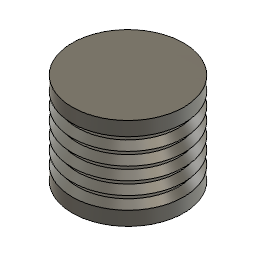
capstan_motor_ed (Autodesk Fusion 360 design; units mm, degrees)
Autodesk Fusion 360 part; units mm, degrees
sketch "Sketch1" plane through (0, 0, 0) normal (0, 1, 0) x (1, 0, 0)
  circle A0 centre (0, 0) radius 10.936
  dimension "d2" = 21.872
  constraint coincident A0.centre origin
  measures "d2" diameter of A0
extrude "Extrude1" add sketch "Sketch1" along normal mid plane 18
sketch "Sketch2" plane through (0, 9, 0) normal (0, 1, 0) x (-1, 0, 0)
  circle A0 centre (0, 0) radius 10.936
  circle A1 centre (0, 0) radius 2.52
  dimension "d7" = 5.04
  constraint coincident A0.centre A1.centre
  measures "d7" diameter of A1
extrude "Extrude2" cut sketch "Sketch2" against normal blind 18 contours A1
sketch "Sketch3" plane through (0, 0, 0) normal (0, 0, 1) x (1, 0, 0)
sketch "Sketch4" plane through (0, 0, 0) normal (0, 0, 1) x (1, 0, 0)
  line L0 (10.936, 9) -> (-10.936, 9)
  line L1 (-10.936, -9) -> (10.936, -9)
  line L2 (10.936, -9) -> (10.936, 9)
  line L3 (10.936, 9) -> (10.936, -9) construction
  line L4 (10.936, 0) -> (10.936, -1.25)
  line L5 (10.936, 0) -> (10.936, 1.25)
  line L6 (10.936, 1.25) -> (9.936, 0)
  line L7 (9.936, 0) -> (10.936, -1.25)
  dimension "d12" = 1.25
  dimension "d13" = 1.25
  dimension "d14" = 1
  constraint coincident L1.end L2.start
  constraint coincident L0.start L2.end
  constraint midpoint L2 L4.start
  constraint perpendicular L1 L4
  constraint perpendicular L1 L5
  measures "d12" distance of L4.start L4.end
  measures "d13" distance of L4.start L5.end
  measures "d14" distance of L4.start L6.end
revolve "Revolve1" cut sketch "Sketch4" angle 360 about axis through (0, 1.75, 0) along (0, 1, 0)
pattern_linear "R-Pattern1" count 5 spacing 2.5 along (0, 1, 0) both ways of "Revolve1"
ref_plane "WorkPlane1" through (0, 7, 0) normal (0, 1, 0) x (0, 0, 1)
sketch "Sketch5" plane through (0, 9, 0) normal (0, 1, 0) x (-1, 0, 0)
  circle A0 centre (0, 0) radius 2.52
  circle A1 centre (0, 0) radius 10.936
  circle A2 centre (0, 0) radius 2.52
  constraint concentric A0 A2
extrude "Extrude3" add sketch "Sketch5" against normal up to surface (2 mm away) contours A0 A2
equation "base_circle_dia = ( ( 10.936 ) * 2 ) * 1 mm"
equation "d2 = base_circle_dia"
equation "base_extrude_one_side = 9 mm"
equation "d4 = base_extrude_one_side"
equation "top_hole = 5.04 mm"
equation "d7 = top_hole"
equation "tri_Rev_side_over_2 = 1.25 mm"
equation "tri_height = 1 mm"
equation "d12 = tri_Rev_side_over_2"
equation "d13 = tri_Rev_side_over_2"
equation "d14 = tri_height"
